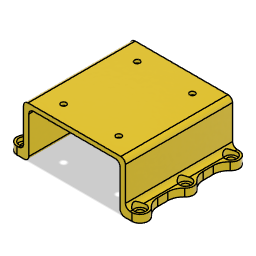
Livox Mount Tassen (Autodesk Fusion 360 design; units mm, degrees)
Autodesk Fusion 360 part; units mm, degrees
note: some values were not read from the file. Chosen so that the rebuilt part matches the saved one: which bodies a step acts on. Set by a fixed rule: which sketch regions a step uses.
sketch "Sketch1" plane through (0, 0, 0) normal (0, 1, 0) x (1, 0, 0)
  line L0 (-37.5, 29.675) -> (-37.5, 0) construction
  line L1 (-37.5, -11.5136) -> (-37.5, -29.675) construction
  line L2 (-37.5, 18.1614) -> (-37.5, 11.5136)
  line L3 (-37.5, -7.5) -> (-37.5, -18.1614)
  line L4 (-37.5, -34.925) -> (-32.25, -34.925)
  line L5 (-32.25, -34.925) -> (-32.25, 34.925)
  line L6 (-32.25, 34.925) -> (-37.5, 34.925)
  arc A0 (-40.9426, 3.9637) -> (-40.9426, -3.9637) centre (-37.5, 0) ccw
  arc A1 (-32.25, 5.3561) -> (-37.5, 7.5) centre (-37.5, 0) ccw construction
  arc A2 (-37.5, -7.5) -> (-32.25, 5.3561) centre (-37.5, 0) ccw construction
  arc A3 (-37.5, 34.925) -> (-40.9426, 25.7113) centre (-37.5, 29.675) ccw
  arc A4 (-37.5, 24.425) -> (-32.25, 29.675) centre (-37.5, 29.675) ccw construction
  arc A5 (-32.25, 29.675) -> (-37.5, 34.925) centre (-37.5, 29.675) ccw construction
  arc A6 (-40.9426, -25.7113) -> (-37.5, -34.925) centre (-37.5, -29.675) ccw
  arc A7 (-37.5, -34.925) -> (-32.25, -29.675) centre (-37.5, -29.675) ccw construction
  arc A8 (-32.25, -29.675) -> (-37.5, -24.425) centre (-37.5, -29.675) ccw construction
  arc A9 (-37.5, 18.1614) -> (-40.9426, 25.7113) centre (-47.5, 18.1614) ccw
  arc A10 (-40.9426, 3.9637) -> (-37.5, 11.5136) centre (-47.5, 11.5136) ccw
  arc A11 (-37.5, -11.5136) -> (-40.9426, -3.9637) centre (-47.5, -11.5136) ccw
  arc A12 (-40.9426, -25.7113) -> (-37.5, -18.1614) centre (-47.5, -18.1614) ccw
  dimension "d1" = 37.5
  dimension "d2" = 29.675
  dimension "d3" = 10.5
  dimension "d4" = 10
  dimension "d5" = 10
  dimension "d6" = 29.675
  dimension "d7" = 7.5
  constraint horizontal origin L0.end
  constraint equal A0 A3
  constraint equal A0 A6
  constraint coincident L0.start A3.centre
  constraint coincident L0.end A0.centre
  constraint vertical L0
  constraint coincident L1.end A6.centre
  constraint parallel L0 L1
  constraint coincident L0 A4.start
  constraint coincident L0 A1.end
  constraint coincident L1 L3.start
  constraint coincident L1 A8.end
  constraint tangent L4 A6
  constraint perpendicular L1 L4
  constraint perpendicular L4 L5
  constraint tangent L6 A3
  constraint horizontal L6
  constraint tangent L5 A3
  constraint coincident L5 A1.start
  constraint concentric A0 A1
  constraint concentric A0 A2
  constraint coincident L5 A4.end
  constraint concentric A3 A4
  constraint concentric A3 A5
  constraint coincident L5 A7.end
  constraint concentric A6 A7
  constraint concentric A6 A8
  constraint coincident A4.start L2
  constraint tangent A3 A9
  constraint tangent L2 A9
  constraint coincident A1.end L2
  constraint tangent A0 A10
  constraint tangent L2 A10
  constraint equal A9 A10
  constraint tangent A0 A11
  constraint tangent L1 A11
  constraint equal A9 A11
  constraint coincident A8.end L3
  constraint tangent A6 A12
  constraint tangent L3 A12
  measures "d1" distance of origin L0.end
  measures "d2" distance of L0.start L0.end
  measures "d3" diameter of A3
  measures "d4" radius of A9
  measures "d5" radius of A12
  measures "d6" distance of L0.end L1.end
  measures "d7" radius of A1
extrude "Extrude1" add sketch "Sketch1" along normal blind 5 makes body 1
sketch "Sketch2" plane through (0, 5, 0) normal (0, 1, 0) x (-1, 0, 0)
  line L0 (37.5, 34.925) -> (32.25, 34.925)
  line L1 (32.25, 34.925) -> (32.25, -34.925) construction
  line L2 (32.25, -34.925) -> (37.5, -34.925)
  arc A0 (37.5, -34.925) -> (40.9426, -25.7113) centre (37.5, -29.675) ccw
  arc A1 (37.5, -18.1614) -> (40.9426, -25.7113) centre (47.5, -18.1614) ccw
  line L3 (37.5, -18.1614) -> (37.5, -11.5136)
  arc A2 (40.9426, -3.9637) -> (37.5, -11.5136) centre (47.5, -11.5136) ccw
  arc A3 (40.9426, -3.9637) -> (40.9426, 3.9637) centre (37.5, 0) ccw
  arc A4 (37.5, 11.5136) -> (40.9426, 3.9637) centre (47.5, 11.5136) ccw
  line L4 (37.5, 11.5136) -> (37.5, 18.1614)
  arc A5 (40.9426, 25.7113) -> (37.5, 18.1614) centre (47.5, 18.1614) ccw
  arc A6 (40.9426, 25.7113) -> (37.5, 34.925) centre (37.5, 29.675) ccw
  arc A7 (40.9426, 25.7113) -> (37.5, 34.925) centre (37.5, 29.675) ccw
  arc A8 (40.9426, 25.7113) -> (37.5, 18.1614) centre (47.5, 18.1614) ccw
  line L5 (37.5, 11.5136) -> (37.5, 18.1614)
  arc A9 (37.5, 11.5136) -> (40.9426, 3.9637) centre (47.5, 11.5136) ccw
  arc A10 (40.9426, -3.9637) -> (40.9426, 3.9637) centre (37.5, 0) ccw
  arc A11 (40.9426, -3.9637) -> (37.5, -11.5136) centre (47.5, -11.5136) ccw
  line L6 (37.5, -18.1614) -> (37.5, -11.5136)
  arc A12 (37.5, -18.1614) -> (40.9426, -25.7113) centre (47.5, -18.1614) ccw
  arc A13 (37.5, -34.925) -> (40.9426, -25.7113) centre (37.5, -29.675) ccw
  line L7 (32.25, -34.925) -> (37.5, -34.925)
  line L8 (32.25, 34.925) -> (32.25, -34.925) construction
  line L9 (37.5, 34.925) -> (32.25, 34.925)
  line L10 (29.75, 34.925) -> (29.75, -34.925)
  line L11 (32.25, 34.925) -> (29.75, 34.925)
  line L12 (29.75, -34.925) -> (32.25, -34.925)
  line L13 (33.25, -34.925) -> (33.25, 34.925)
  dimension "d33" = 2.5
  dimension "d36" = 1
  constraint coincident L7 L10.end
  constraint coincident L9 L10.start
  constraint coincident L0.end L1.start
  constraint coincident L1.end L2.start
  constraint coincident L2 L13.start
  constraint coincident L9 L13.end
  constraint perpendicular L9 L13
  measures "d33" distance of L8 L10
  measures "d36" distance of L8 L13
extrude "Extrude2" add sketch "Sketch2" along normal blind 25 and the other way blind 5 contours L0 L2 L7 L9 L10 L11 L12 L13 bodies 1
mirror "Mirror1" about plane through (0, 0, 0) normal (1, 0, 0) of bodies 1 makes body 2
sketch "Sketch3" plane through (0, 30, 0) normal (0, 1, 0) x (-1, 0, 0)
  line L0 (33.25, -34.925) -> (-33.25, -34.925)
  line L1 (-33.25, -34.925) -> (-33.25, 34.925)
  line L2 (-33.25, 34.925) -> (33.25, 34.925)
  line L3 (33.25, 34.925) -> (33.25, -34.925)
  line L4 (29.75, 34.925) -> (29.75, -34.925) construction
  line L5 (-29.75, -34.925) -> (-29.75, 34.925) construction
  line L6 (33.25, 34.925) -> (29.75, 34.925)
  line L7 (29.75, -34.925) -> (33.25, -34.925)
  line L8 (-33.25, -34.925) -> (-29.75, -34.925)
  line L9 (-29.75, 34.925) -> (-33.25, 34.925)
  line L10 (33.25, -34.925) -> (33.25, 34.925)
  line L11 (-33.25, 34.925) -> (-33.25, -34.925)
  constraint horizontal L0
  constraint vertical L1
  constraint horizontal L2
  constraint vertical L3
  constraint coincident L2 L4.start
  constraint coincident L0 L5.start
  constraint coincident L3 L0.start
  constraint coincident L1 L0.end
extrude "Extrude3" add sketch "Sketch3" along normal blind 3 bodies 1 2
sketch "Sketch5" plane through (0, 5, 0) normal (0, 1, 0) x (-1, 0, 0)
  line L0 (-33.25, 34.925) -> (-37.5, 34.925)
  arc A0 (-37.5, 34.925) -> (-40.9426, 25.7113) centre (-37.5, 29.675) ccw
  arc A1 (-37.5, 18.1614) -> (-40.9426, 25.7113) centre (-47.5, 18.1614) ccw
  line L1 (-37.5, 18.1614) -> (-37.5, 11.5136)
  arc A2 (-40.9426, 3.9637) -> (-37.5, 11.5136) centre (-47.5, 11.5136) ccw
  arc A3 (-40.9426, 3.9637) -> (-40.9426, -3.9637) centre (-37.5, 0) ccw
  arc A4 (-37.5, -11.5136) -> (-40.9426, -3.9637) centre (-47.5, -11.5136) ccw
  line L2 (-37.5, -11.5136) -> (-37.5, -18.1614)
  arc A5 (-40.9426, -25.7113) -> (-37.5, -18.1614) centre (-47.5, -18.1614) ccw
  arc A6 (-40.9426, -25.7113) -> (-37.5, -34.925) centre (-37.5, -29.675) ccw
  line L3 (-37.5, -34.925) -> (-33.25, -34.925)
  arc A7 (40.9426, 25.7113) -> (37.5, 34.925) centre (37.5, 29.675) ccw
  arc A8 (40.9426, -3.9637) -> (40.9426, 3.9637) centre (37.5, 0) ccw
  arc A9 (37.5, -34.925) -> (40.9426, -25.7113) centre (37.5, -29.675) ccw
  arc A10 (-40.9426, -25.7113) -> (-37.5, -34.925) centre (-37.5, -29.675) ccw
  arc A11 (-40.9426, 3.9637) -> (-40.9426, -3.9637) centre (-37.5, 0) ccw
  arc A12 (-37.5, 34.925) -> (-40.9426, 25.7113) centre (-37.5, 29.675) ccw
  line L4 (-33.25, -34.925) -> (-33.25, 34.925)
hole "Hole2" at (-37.5, 5, -29.675) at (-37.5, 5, 0) at (-37.5, 5, 29.675) at (37.5, 5, -29.675) at (37.5, 5, 0) at (37.5, 5, 29.675) direction (0, -1, 0) diameter 4.5 depth 20 tip angle 118 counterbore diameter 7.75 counterbore depth 2.5 bodies 1
fillet "Fillet1" radius 3 8 edges at (33.25, 5, 0) (-33.25, 5, 0) (-33.25, 33, 0) (33.25, 33, 0) (29.75, 0, 0) (29.75, 30, 0) (-29.75, 30, 0) (-29.75, 0, 0) on bodies 1
sketch "Sketch4" plane through (0, 30, 0) normal (0, -1, 0) x (1, 0, 0)
  line L0 (-26.75, -34.925) -> (26.75, -34.925)
  line L1 (26.75, 34.925) -> (-26.75, 34.925)
  line L2 (18, 24) -> (-18, 24) construction
  line L3 (-18, 24) -> (-18, -24) construction
  line L4 (-18, -24) -> (18, -24) construction
  line L5 (18, -24) -> (18, 24) construction
  line L6 (18, 24) -> (-18, -24) construction
  line L7 (-18, 24) -> (18, -24) construction
  circle A0 centre (-18, 24) radius 5
  circle A1 centre (18, 24) radius 5
  circle A2 centre (-18, -24) radius 5
  circle A3 centre (18, -24) radius 5
  line L8 (-26.75, 34.925) -> (-26.75, -34.925)
  line L9 (26.75, -34.925) -> (26.75, 34.925)
  dimension "d20" = 36
  dimension "d21" = 48
  dimension "d22" = 10
  constraint horizontal L2
  constraint perpendicular L2 L3
  constraint parallel L2 L4
  constraint parallel L3 L5
  constraint coincident L6 origin
  constraint coincident L7 origin
  constraint coincident L2.end L3.start
  constraint coincident L2.start L5.end
  constraint coincident L3.end L4.start
  constraint coincident L4.end L5.start
  constraint equal A0 A2
  constraint equal A2 A3
  constraint equal A1 A3
  measures "d20" distance of L2.start L2.end
  measures "d21" distance of L2.start L4.end
  measures "d22" diameter of A0
hole "Hole1" at (-18, 30, 24) at (18, 30, 24) at (18, 30, -24) at (-18, 30, -24) direction (0, 1, 0) diameter 3.5 depth 20 tip angle 118 counterbore diameter 5.75 counterbore depth 1 bodies 1
sketch "Sketch6" plane through (0, 0, 0) normal (1, 0, 0) x (0, 0, -1)
  line L0 (34.925, 30) -> (-34.925, 30)
  line L1 (-34.925, 30) -> (-34.925, 8)
  line L2 (-34.925, 8) -> (34.925, 8)
  line L3 (34.925, 8) -> (34.925, 30)
  line L4 (-34.925, 8) -> (34.925, 30) construction
  line L5 (-34.4744, 6.5693) -> (35.3756, 28.5693)
  line L6 (-35.3756, 9.4307) -> (34.4744, 31.4307)
  line L7 (32.925, 8) -> (32.925, 30)
  line L8 (-32.925, 30) -> (-32.925, 8)
  dimension "d37" = 1.5
  dimension "d38" = -1.5
  dimension "d39" = -2
  dimension "d40" = -2
  constraint coincident L1.end L2.start
  constraint coincident L0.start L3.end
extrude "Extrude4" add sketch "Sketch6" along normal mid plane 90 separate body contours L0 L6 L8 | L2 L5 L7 makes body 3 at (-15, 16.8017, 11.9727) makes body 4 at (-15, 14.5991, 8.9796)
fillet "Fillet2" radius 2 2 edges at (0, 30, -29.9319) (0, 8, 29.9319) on bodies 3 4
fillet "Fillet2" radius 5 2 edges at (0, 30, 32.925) (0, 8, -32.925) on bodies 3 4
fillet "Fillet2" radius 3 2 edges at (0, 10.2026, 32.925) (0, 27.7974, -32.925) on bodies 3 4
sketch "Sketch7" plane through (-45, 0, 0) normal (-1, 0, 0) x (0, 0, 1)
  arc A0 (-29.0238, 26.5687) -> (-32.925, 23.7073) centre (-29.925, 23.7073) ccw
  line L0 (-32.925, 23.7073) -> (-32.925, 13)
  arc A1 (-32.925, 13) -> (-27.925, 8) centre (-27.925, 13) ccw
  line L1 (-27.925, 8) -> (16.9243, 8)
  arc A2 (16.9243, 8) -> (17.5252, 11.9076) centre (16.9243, 10) ccw
  line L2 (17.5252, 11.9076) -> (-29.0238, 26.5687)
  line L3 (34.925, 0) -> (34.925, 5)
  line L4 (34.925, 8) -> (34.925, 5)
  line L5 (34.925, 8) -> (34.925, 30)
  line L6 (34.925, 33) -> (34.925, 30)
  line L7 (-34.925, 0) -> (-25.7113, 0)
  line L8 (-18.1614, 0) -> (-25.7113, 0)
  line L9 (-18.1614, 0) -> (-11.5136, 0)
  line L10 (-3.9637, 0) -> (-11.5136, 0)
  line L11 (-3.9637, 0) -> (3.9637, 0)
  line L12 (11.5136, 0) -> (3.9637, 0)
  line L13 (11.5136, 0) -> (18.1614, 0)
  line L14 (25.7113, 0) -> (18.1614, 0)
  line L15 (25.7113, 0) -> (34.925, 0)
  line L16 (-34.925, 30) -> (-34.925, 33)
  line L17 (-34.925, 30) -> (-34.925, 8)
  line L18 (-34.925, 5) -> (-34.925, 8)
  line L19 (-34.925, 0) -> (-34.925, 5)
  line L20 (-34.925, 33) -> (34.925, 33)
  line L21 (-39.925, 33) -> (39.925, 33)
  line L22 (39.925, 33) -> (39.925, 0)
  line L23 (39.925, 0) -> (-39.925, 0)
  line L24 (-39.925, 0) -> (-39.925, 33)
  dimension "d70" = 5
  dimension "d71" = 5
  constraint horizontal L21
  constraint vertical L22
  constraint horizontal L23
  constraint vertical L24
  constraint coincident L16.end L21
  constraint coincident L7.start L23
  measures "d70" distance of L17 L24
  measures "d71" distance of L5 L22
extrude "Extrude5" add sketch "Sketch7" along normal blind 3 separate body contours A0 L0 A1 L1 A2 L2 | L3 L4 L5 L6 L7 L8 L9 L10 L11 L12 L13 L14 L15 L16 L17 L18 L19 L20 L21 L23 | L3 L4 L5 L6 L21 L22 L23 | L16 L17 L18 L19 L21 L23 L24 makes body 5
mirror "Mirror2" about plane through (0, 0, 0) normal (1, 0, 0) of bodies 5 makes body 6
sketch "Sketch8" plane through (0, 0, 34.925) normal (0, 0, 1) x (1, 0, 0)
  line L0 (-48, 33) -> (48, 33)
  line L1 (48, 33) -> (48, 0)
  line L2 (48, 0) -> (-48, 0)
  line L3 (-48, 0) -> (-48, 33)
  line L4 (-45, 0) -> (-45, 33)
  line L5 (-45, 33) -> (-48, 33)
  line L6 (-48, 33) -> (-48, 0)
  line L7 (-48, 0) -> (-45, 0)
  arc A0 (-32.75, 0) -> (-29.75, 3) centre (-32.75, 3) ccw
  line L8 (-29.75, 3) -> (-29.75, 27)
  arc A1 (-26.75, 30) -> (-29.75, 27) centre (-26.75, 27) ccw
  line L9 (-26.75, 30) -> (26.75, 30)
  arc A2 (29.75, 27) -> (26.75, 30) centre (26.75, 27) ccw
  line L10 (29.75, 27) -> (29.75, 3)
  arc A3 (29.75, 3) -> (32.75, 0) centre (32.75, 3) ccw
  line L11 (32.75, 0) -> (37.5, 0)
  line L12 (37.5, 0) -> (37.5, 5)
  line L13 (37.5, 5) -> (36.25, 5)
  arc A4 (33.25, 8) -> (36.25, 5) centre (36.25, 8) ccw
  line L14 (33.25, 8) -> (33.25, 30)
  arc A5 (33.25, 30) -> (30.25, 33) centre (30.25, 30) ccw
  line L15 (30.25, 33) -> (-30.25, 33)
  arc A6 (-30.25, 33) -> (-33.25, 30) centre (-30.25, 30) ccw
  line L16 (-33.25, 30) -> (-33.25, 8)
  arc A7 (-36.25, 5) -> (-33.25, 8) centre (-36.25, 8) ccw
  line L17 (-36.25, 5) -> (-37.5, 5)
  line L18 (-37.5, 5) -> (-37.5, 0)
  line L19 (-37.5, 0) -> (-32.75, 0)
  constraint horizontal L0
  constraint vertical L1
  constraint horizontal L2
  constraint vertical L3
  constraint coincident L3 L0.start
extrude "Extrude6" add sketch "Sketch8" along normal blind 3 from surface at 5 separate body makes body 7
sketch "Sketch9" plane through (0, 33, 0) normal (0, 1, 0) x (-1, 0, 0)
  circle A0 centre (-18, -24) radius 1.75
  circle A1 centre (18, 24) radius 1.75
  circle A2 centre (-18, 24) radius 1.75
  circle A3 centre (18, -24) radius 1.75
  line L0 (-30.25, 34.925) -> (-30.25, -34.925)
  line L1 (-30.25, -34.925) -> (30.25, -34.925)
  line L2 (30.25, -34.925) -> (30.25, 34.925)
  line L3 (30.25, 34.925) -> (-30.25, 34.925)
  line L4 (27.25, -31.925) -> (27.25, 31.925)
  line L5 (27.25, 31.925) -> (-27.25, 31.925)
  line L6 (-27.25, 31.925) -> (-27.25, -31.925)
  line L7 (-27.25, -31.925) -> (27.25, -31.925)
  line L8 (-23.9437, -31.925) -> (23.9438, 31.925) construction
  line L9 (23.9438, -31.925) -> (-23.9438, 31.925) construction
  line L10 (-20.1937, -31.925) -> (27.6938, 31.925)
  line L11 (-27.6938, -31.925) -> (20.1938, 31.925)
  line L12 (27.6937, -31.925) -> (-20.1938, 31.925)
  line L13 (20.1937, -31.925) -> (-27.6938, 31.925)
  dimension "d55" = -3
  dimension "d56" = 3
  dimension "d57" = -3
  dimension "d58" = 3
  dimension "d59" = -3
  constraint coincident A2.centre L9
  constraint coincident A3.centre L9
  constraint coincident L7 L9.start
  constraint coincident L5 L9.end
  constraint coincident A0.centre L8
  constraint coincident A1.centre L8
  constraint coincident L7 L8.start
  constraint coincident L5 L8.end
  constraint coincident L7 L12.start
  constraint coincident L7 L13.start
  constraint coincident L7 L10.start
  constraint coincident L7 L11.start
  constraint coincident L5 L13.end
  constraint coincident L5 L12.end
  constraint coincident L5 L11.end
  constraint coincident L5 L10.end
extrude "Extrude7" add sketch "Sketch9" along normal blind 10 and the other way blind 20 separate body contours L4 L10 L12 | L7 L10 L13 | L5 L11 L12 | L6 L11 L13 makes body 8 at (6.7313, 23, -31.925) makes body 9 at (27.25, 23, 10.4444) makes body 10 at (6.7313, 33, 31.925) makes body 11 at (-27.25, 33, 10.4444)
fillet "Fillet3" radius 3 8 edges at (-20.1937, 28, -31.925) (20.1937, 28, -31.925) (27.25, 28, -31.3333) (27.25, 28, 31.3333) (20.1938, 28, 31.925) (-20.1938, 28, 31.925) (-27.25, 28, 31.3333) (-27.25, 28, -31.3333) on bodies 8 9 10 11
fillet "Fillet3" radius 3 4 edges at (0, 28, -5) (3.75, 28, 0) (0, 28, 5) (-3.75, 28, 0) on bodies 8 9 10 11
mirror "Mirror3" about plane through (0, 0, 0) normal (0, 0, 1) of bodies 7 makes body 12
combine "Combine1" operation add target body 3 tool bodies 4 5 6 7 9 8 11 10 12
delete_body "RemoveBody1" bodies 3
equation "d1 = ( ( 75 / 2 ) * 1 mm )"
equation "d3 = ( 5.25 * 2 ) * 1 mm"
equation "d6 = d2"
equation "d57 = -d56"
equation "d58 = d56"
equation "d59 = d57"
